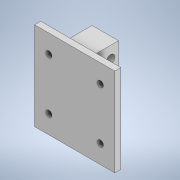
# Autodesk Inventor part: bearing support
Saved by Autodesk Inventor 2022 (Build 260153000, 153)
## iProperties
Created: 2022-02-16
Part Number: bearing support
Material: Generic
Document SubType Name: Modeling
Designer: erasm
Density: 1 g/cm^3
Appearance: Default
Author: erasm
Autodesk Inventor part; units mm, degrees
ref_plane "YZ Plane" through (0, 0, 0) normal (1, 0, 0) x (0, 1, 0)
ref_plane "XZ Plane" through (0, 0, 0) normal (0, 1, 0) x (-1, 0, 0)
ref_plane "XY Plane" through (0, 0, 0) normal (0, 0, 1) x (1, 0, 0)
sketch "Sketch1" plane through (0, 0, 0) normal (0, 0, 1) x (1, 0, 0)
  line L0 (0, 0) -> (36.8826, 0) projected
  line L1 (36.8826, 0) -> (36.8826, 40) projected
  line L2 (0, 40) -> (36.8826, 40) projected
  line L3 (0, 0) -> (0, 40) projected
  line L4 (-21.6348, 40) -> (-58.5174, 40) projected
  line L5 (-58.5174, 40) -> (-58.5174, 0) projected
  line L6 (-21.6348, 0) -> (-58.5174, 0) projected
  line L7 (-21.6348, 40) -> (-21.6348, 0) projected
  line L8 (-21.6348, -8) -> (-58.5174, -8) projected
  line L9 (-58.5174, -8) -> (-58.5174, -48) projected
  line L10 (-21.6348, -48) -> (-58.5174, -48) projected
  line L11 (-21.6348, -8) -> (-21.6348, -48) projected
  line L12 (0, -48) -> (36.8826, -48) projected
  line L13 (36.8826, -48) -> (36.8826, -8) projected
  line L14 (0, -8) -> (36.8826, -8) projected
  line L15 (0, -48) -> (0, -8) projected
  line L16 (21.8826, 32) -> (-43.5174, 32)
  line L17 (-43.5174, 32) -> (-43.5174, -40)
  line L18 (-43.5174, -40) -> (21.8826, -40)
  line L19 (21.8826, -40) -> (21.8826, 32)
  dimension "d0" = 8
  dimension "d1" = 8
  dimension "d2" = 15
  dimension "d3" = 15
  constraints: 8 end point, 2 parallel, 1 horizontal, 1 perpendicular
  measures "d0" distance between parallel lines of L2 L16
  measures "d1" distance between parallel lines of L12 L18
  measures "d2" distance between parallel lines of L19 L13
  measures "d3" distance between parallel lines of L9 L17
extrude "Extrusion1" add sketch "Sketch1" along normal blind 5 contours L3 L16 L19 L0 | L0 L19 L14 L15 L18 L11 L8 L17 L6 L7 L16 L3 | L19 L18 L15 L14 | L7 L6 L17 L16 | L18 L17 L8 L11
sketch "Sketch2" plane through (0, 0, 0) normal (0, 0, -1) x (-1, 0, 0)
  line L0 (0, -48) -> (-36.8826, -48) projected
  line L1 (-36.8826, -48) -> (-36.8826, -8) projected
  line L2 (0, -8) -> (-36.8826, -8) projected
  line L3 (0, -48) -> (0, -8) projected
  line L4 (0, 0) -> (-36.8826, 0) projected
  line L5 (-36.8826, 0) -> (-36.8826, 40) projected
  line L6 (0, 40) -> (-36.8826, 40) projected
  line L7 (0, 0) -> (0, 40) projected
  line L8 (21.6348, 40) -> (58.5174, 40) projected
  line L9 (58.5174, 40) -> (58.5174, 0) projected
  line L10 (21.6348, 0) -> (58.5174, 0) projected
  line L11 (21.6348, 40) -> (21.6348, 0) projected
  line L12 (21.6348, -8) -> (58.5174, -8) projected
  line L13 (58.5174, -8) -> (58.5174, -48) projected
  line L14 (21.6348, -48) -> (58.5174, -48) projected
  line L15 (21.6348, -8) -> (21.6348, -48) projected
  line L16 (0, -38) -> (21.6348, -38)
  line L17 (21.6348, -38) -> (21.6348, -18)
  line L18 (21.6348, -18) -> (0, -18)
  line L19 (0, -18) -> (0, -38)
  line L20 (0, 10) -> (21.6348, 10)
  line L21 (21.6348, 10) -> (21.6348, 30)
  line L22 (21.6348, 30) -> (0, 30)
  line L23 (0, 30) -> (0, 10)
  point P0 (0, 30)
  point P1 (0, -18)
  dimension "d6" = 20
  dimension "d7" = 20
  dimension "d8" = 10
  dimension "d9" = 10
  constraints: 16 end point, 4 parallel, 4 point on line, 2 horizontal, 2 perpendicular
  measures "d6" distance between parallel lines of L18 L16
  measures "d7" distance between parallel lines of L22 L20
  measures "d8" distance between parallel lines of L2 L18
  measures "d9" distance between parallel lines of L20 L4
extrude "Extrusion2" add sketch "Sketch2" along normal blind 20 contours L3 L18 L15 L16 | L7 L22 L11 L20
sketch "Sketch3" plane through (0, 0, 5) normal (0, 0, 1) x (1, 0, 0)
  circle A0 centre (10.1826, 17) radius 2.5
  circle A1 centre (-31.8174, 17) radius 2.5
  circle A2 centre (10.1826, -25) radius 2.5
  circle A3 centre (-31.8174, -25) radius 2.5
  line L0 (21.8826, -40) -> (21.8826, 32) projected
  line L1 (-43.5174, 32) -> (-43.5174, -40) projected
  line L2 (10.1826, 17) -> (-31.8174, 17)
  line L3 (10.1826, -25) -> (-31.8174, -25)
  line L4 (21.8826, 32) -> (-43.5174, 32) projected
  line L5 (-43.5174, -40) -> (21.8826, -40) projected
  point P0 (0, 0)
  point P1 (-10.8174, 17)
  point P2 (-10.8174, 32)
  point P3 (-10.8174, -25)
  point P4 (-10.8174, -40)
  dimension "d12" = 5
  dimension "d13" = 5
  dimension "d14" = 5
  dimension "d15" = 5
  dimension "d16" = 42
  dimension "d17" = 42
  dimension "d18" = 15
  dimension "d19" = 15
  constraints: 4 centre point, 4 end point, 4 midpoint, 2 horizontal, 2 vertical alignment, 1 coincident
  measures "d12" diameter of A0
  measures "d13" diameter of A1
  measures "d14" diameter of A2
  measures "d15" diameter of A3
  measures "d16" distance of L2.end L2.start
  measures "d17" distance of A3.centre L3.start
  measures "d18" distance from line of L4 L2.start
  measures "d19" distance from line of L5 L3.start
extrude "Extrusion3" cut sketch "Sketch3" against normal through all contours A0 | A1 | A2 | A3
sketch "Sketch4" plane through (0, -38, 0) normal (1, 0, 0) x (0, 0, -1)
  arc A0 (2.5, 58) -> (5, 53.6699) centre (7.5, 58) ccw projected
  arc A1 (5, 53.6699) -> (10, 53.6699) centre (7.5, 58) ccw projected
  arc A2 (10, 53.6699) -> (12.5, 58) centre (7.5, 58) ccw projected
  arc A3 (12.5, 58) -> (10, 62.3301) centre (7.5, 58) ccw projected
  arc A4 (10, 62.3301) -> (5, 62.3301) centre (7.5, 58) ccw projected
  arc A5 (5, 62.3301) -> (2.5, 58) centre (7.5, 58) ccw projected
  circle A6 centre (7.5, 58) radius 3.1 projected
  arc A7 (2.3201, 9.9991) -> (4.8201, 5.669) centre (7.3201, 9.9991) ccw projected
  arc A8 (4.8201, 5.669) -> (9.8201, 5.669) centre (7.3201, 9.9991) ccw projected
  arc A9 (9.8201, 5.669) -> (12.3201, 9.9991) centre (7.3201, 9.9991) ccw projected
  arc A10 (12.3201, 9.9991) -> (9.8201, 14.3292) centre (7.3201, 9.9991) ccw projected
  arc A11 (9.8201, 14.3292) -> (4.8201, 14.3292) centre (7.3201, 9.9991) ccw projected
  arc A12 (4.8201, 14.3292) -> (2.3201, 9.9991) centre (7.3201, 9.9991) ccw projected
  circle A13 centre (7.3201, 9.9991) radius 3.1 projected
  circle A14 centre (13.5, 58) radius 3.5
  circle A15 centre (13.5, 9.9991) radius 3.5
  line L0 (0, -2) -> (0, 70) projected
  point P0 (0, 38)
  dimension "d24" = 7
  dimension "d25" = 7
  dimension "d26" = 10
  dimension "d27" = 10
  constraints: 2 centre point, 2 horizontal alignment
  measures "d24" diameter of A14
  measures "d25" diameter of A15
  measures "d26" distance edge to line of A14 L0
  measures "d27" distance edge to line of A15 L0
extrude "Extrusion5" cut sketch "Sketch4" against normal through all contours A14 A6 A3 A2 | A2 A3 A14 | A14 A6 | A15 A13 A10 A9 | A9 A10 A15 | A15 A13 picked at (10.2115, 57.6094) picked at (10.1547, 9.9991)
body "Solid1"
